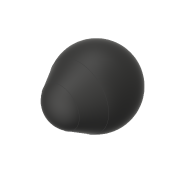
# Autodesk Inventor part: PolyformA7Buoy_Black
Saved by Autodesk Inventor 2019.4 (Build 234330000, 330)
## iProperties
Created: 2021-05-16
Part Number: PolyformA7Buoy_Black
Material: 一般
Document SubType Name: Modeling
Designer: Sanada Tatsuya
Density: 1 g/cm^3
Appearance: 滑らか - 黒
Author: Sanada Tatsuya
Autodesk Inventor part; units mm, degrees
ref_plane "YZ Plane" through (0, 0, 0) normal (1, 0, 0) x (0, 1, 0)
ref_plane "XZ Plane" through (0, 0, 0) normal (0, 1, 0) x (-1, 0, 0)
ref_plane "XY Plane" through (0, 0, 0) normal (0, 0, 1) x (1, 0, 0)
sketch "スケッチ1" plane through (0, 0, 0) normal (0, 1, 0) x (-1, 0, 0)
  line L0 (0, 0) -> (0, 948.6182)
  arc A0 (-476.314, 275) -> (0, -550) centre (0, 0) ccw
  line L1 (0, 750) -> (0, -550)
  line L2 (-550, 439.5467) -> (-550, -285.6332) construction
  line L3 (574.7081, 870) -> (-1081.4689, 870) construction
  line L4 (-303.1089, 575) -> (-476.314, 275)
  arc A1 (0, 750) -> (-303.1089, 575) centre (0, 400) ccw
  dimension "d0" = 1100
  dimension "d1" = 1420
  dimension "d2" = 350
  dimension "d3" = 30
  constraints: 10 end point, 4 point on circle, 3 tangent, 3 vertical, 2 centre point, 2 point on line, 1 coincident, 1 collinear, 1 horizontal
  measures "d0" diameter of L2 L0
  measures "d1" distance from line of L1.end L3
  measures "d2" radius of A1
  measures "d3" angle of L4 L1
revolve "回転1" add sketch "スケッチ1" angle 360 about axis through (0, 0, 0) along (0, 0, 1)
